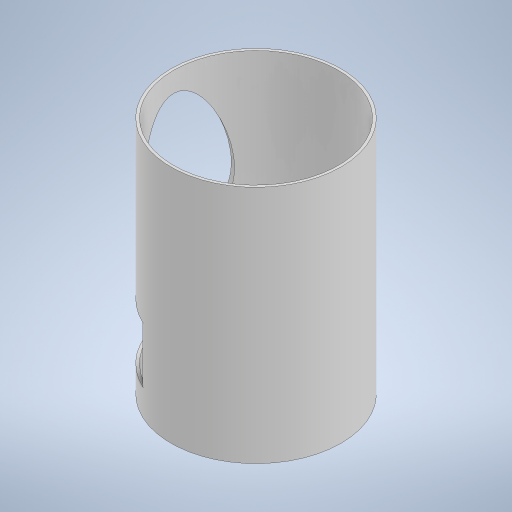
# Autodesk Inventor part: Insulation Shaft
Saved by Autodesk Inventor 2024.3 (Build 283343000, 343)
## iProperties
Created: 2025-03-01
Part Number: Insulation Shaft
Material: Generic
Document SubType Name: Modeling
Designer: ajclo
Density: 1 g/cm^3
Appearance: Default
Author: ajclo
Autodesk Inventor part; units mm, degrees
ref_plane "XZ Plane" through (0, 0, 0) normal (0, 1, 0) x (-1, 0, 0)
ref_plane "XY Plane" through (0, 0, 0) normal (0, 0, 1) x (1, 0, 0)
sketch "Sketch1" plane through (0, 0, 0) normal (0, 1, 0) x (-1, 0, 0)
  circle A0 centre (0, 0) radius 62
  circle A1 centre (0, 0) radius 64
  dimension "d0" = 2
  dimension "d1" = 128
  constraints: 2 centre point, 2 coincident
  measures "d0" radial gap between concentric circles of A1 A0
  measures "d1" diameter of A1
extrude "Extrusion1" add sketch "Sketch1" along normal blind 180
sketch "Sketch2" plane through (0, 0, 0) normal (1, 0, 0) x (0, 1, 0)
  line L0 (20, 58) -> (62, 58)
  line L1 (62, 58) -> (62, -58)
  line L2 (62, -58) -> (20, -58)
  line L3 (20, -58) -> (20, 58)
  line L4 (0, -64) -> (0, 64) projected
  point P0 (0, 0)
  point P1 (0, 0)
  point P2 (41, 58)
  dimension "d4" = 42
  dimension "d5" = 116
  dimension "d6" = 20
  dimension "d7" = 58
  constraints: 8 end point, 2 midpoint, 2 parallel, 1 horizontal, 1 perpendicular
  measures "d4" distance of L1.end L2.end
  measures "d5" distance of L0.end L1.end
  measures "d6" distance between parallel lines of L4 L3
  measures "d7" vertical distance of point (0, 0) point (41, 58)
extrude "Extrusion2" cut sketch "Sketch2" against normal through all
sketch "Sketch3" plane through (0, 0, 0) normal (1, 0, 0) x (0, 1, 0)
  line L0 (110, -32.8663) -> (110, 39.5028)
  line L1 (0, -64) -> (0, 64) projected
  point P0 (0, 0)
  point P1 (110, 3.3182)
  dimension "d10" = 110
  constraints: 2 end point, 1 midpoint, 1 vertical
  measures "d10" distance from line of L1 point (110, 3.318)
ref_plane "Work Plane1" through (0, 110, -32.8663) normal (-0.7071, 0.7071, 0) x (0, 0, 1)
sketch "Sketch4" plane through (0, 110, -32.8663) normal (-0.7071, 0.7071, 0) x (0, 0, 1)
  circle A0 centre (32.8663, -40) radius 35
  line L0 (0, 0) -> (72.3691, 0) construction
  point P0 (32.8663, -77.7817)
  point P1 (36.1845, 0)
  dimension "d12" = 70
  dimension "d15" = 40
  constraints: 1 centre point
  measures "d12" diameter of A0
  measures "d15" vertical distance of point (36.185, 0) A0.centre
extrude "Extrusion3" cut sketch "Sketch4" along normal through all
body "Solid1"
